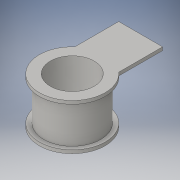
# Autodesk Inventor part: Generator placement
Saved by Autodesk Inventor 2016 SP1 (Build 200210100, 210)
## iProperties
Created: 2016-02-19
Part Number: Generator placement
Material: Generic
Document SubType Name: Modeling
Designer: Tore Den Store
Density: 1 g/cm^3
Appearance: Default
Author: Tore Den Store
Autodesk Inventor part; units mm, degrees
ref_plane "YZ Plane" through (0, 0, 0) normal (1, 0, 0) x (0, 1, 0)
ref_plane "XZ Plane" through (0, 0, 0) normal (0, 1, 0) x (-1, 0, 0)
sketch "Sketch1" plane through (0, 0, 0) normal (0, 0, 1) x (1, 0, 0)
  circle A0 centre (0, 0) radius 130
  dimension "d0" = 260
  constraints: 1 centre point, 1 coincident
  measures "d0" diameter of A0
extrude "Extrusion1" add sketch "Sketch1" along normal blind 180
sketch "Sketch2" plane through (0, 0, 180) normal (0, 0, 1) x (1, 0, 0)
  circle A0 centre (0, 0) radius 150
  dimension "d3" = 300
  constraints: 1 centre point, 1 coincident
  measures "d3" diameter of A0
extrude "Extrusion2" add sketch "Sketch2" along normal blind 15
ref_plane "Work Plane3" through (0, 0, 90) normal (0, 0, -1) x (-1, 0, 0)
mirror "Mirror2" about plane through (0, 0, 90) normal (0, 0, -1) of "Extrusion2"
hole "Hole2" at (0, 0, 195) direction (0, 0, -1) diameter 200 end through all
sketch "Sketch6" plane through (0, 0, 195) normal (0, 0, 1) x (1, 0, 0)
  line L0 (-100, 111.8034) -> (100, 111.8034) construction
  line L1 (100, 111.8034) -> (100, 311.8034)
  line L2 (100, 311.8034) -> (-100, 311.8034)
  line L3 (-100, 311.8034) -> (-100, 111.8034)
  circle A0 centre (0, 0) radius 150 projected
  dimension "d36" = 200
  dimension "d37" = 200
  constraints: 8 end point, 2 parallel, 2 point on circle, 1 horizontal, 1 perpendicular
  measures "d36" distance of L2.end L1.end
  measures "d37" distance of L1.end L0.end
extrude "Extrusion6" add sketch "Sketch6" against normal blind 15 contours A0 L3 L2 L1
body "Solid1"
